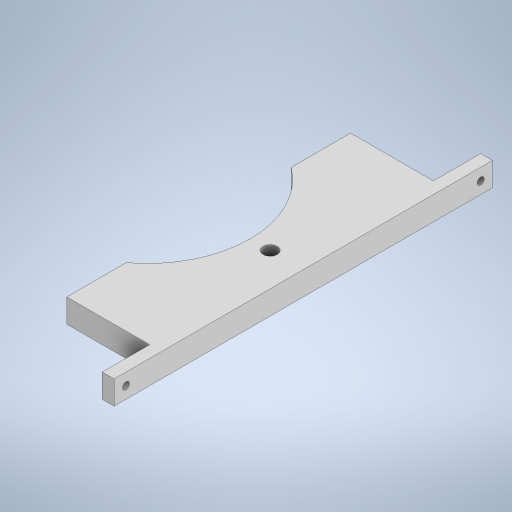
# Autodesk Inventor part: Мотор стенка
Saved by Autodesk Inventor 2023 (Build 270158000, 158)
## iProperties
Created: 2022-05-23
Part Number: Мотор стенка
Material: Типовые
Document SubType Name: Modeling
Designer: User
Density: 1 g/cm^3
Appearance: По умолчанию
Author: User
Autodesk Inventor part; units mm, degrees
ref_plane "YZ Plane" through (0, 0, 0) normal (1, 0, 0) x (0, 1, 0)
ref_plane "XZ Plane" through (0, 0, 0) normal (0, 1, 0) x (-1, 0, 0)
ref_plane "XY Plane" through (0, 0, 0) normal (0, 0, 1) x (1, 0, 0)
sketch "Эскиз1" plane through (0, 0, 0) normal (0, 1, 0) x (-1, 0, 0)
  line L0 (0, 0) -> (130, 0)
  line L1 (130, 0) -> (130, -120)
  line L2 (130, -120) -> (0, -120)
  line L3 (0, -120) -> (0, 0)
  line L4 (0, -60) -> (66, -60)
  circle A0 centre (66, -60) radius 43.5
  line L5 (130, 0) -> (90, 0)
  line L6 (90, -120) -> (130, -120)
  line L7 (130, -120) -> (130, 0)
  line L8 (0, 0) -> (40, 0)
  line L9 (40, 0) -> (40, -120)
  line L10 (40, -120) -> (0, -120)
  line L11 (0, -120) -> (0, 0)
  line L12 (0, 0) -> (0, 20)
  line L13 (0, 20) -> (5, 20)
  line L14 (5, 20) -> (5, -140)
  line L15 (5, -140) -> (0, -140)
  line L16 (0, -140) -> (0, -120)
  circle A1 centre (66, -60) radius 52
  circle A2 centre (14, -60) radius 3
  point P0 (40, -25.1252)
  point P1 (40, -94.8748)
  point P2 (5, -120)
  point P3 (5, 0)
  dimension "d34" = 104
  dimension "d0" = 130
  dimension "d1" = 120
  dimension "d2" = 66
  dimension "d16" = 87
  dimension "d20" = 40
  dimension "d21" = 20
  dimension "d22" = 5
  dimension "d23" = 160
  dimension "d35" = 6
  constraints: 34 end point, 6 perpendicular, 5 parallel, 4 horizontal, 3 point on line, 2 centre point, 1 coincident, 1 horizontal alignment, 1 midpoint, 1 vertical, 2 other
  measures "d0" distance of L1.end L2.end
  measures "d1" distance of L0.end L1.end
  measures "d2" distance of L4.start L4.end
  measures "d16" diameter of A0
  measures "d20" distance of L9.end L10.end
  measures "d21" distance of L0.start L12.end
  measures "d22" distance of L12.end L13.end
  measures "d23" distance of L13.end L14.end
  measures "d35" diameter of A2
extrude "Выдавливание1" add sketch "Эскиз1" along normal blind 10 contours L9 A1 A2 L4 L14 L0 | L14 L4 L3 L0 | L0 L12 L13 L14 | L9 A0 L4 A2 A1 | L14 L2 L3 L4 | L4 A2 A1 L9 L2 L14 | L14 L15 L16 L2 | A0 L9 A1 A2 L4
sketch "Эскиз2" plane through (-5, 0, 0) normal (-1, 0, 0) x (0, 0, 1)
  line L0 (20, 0) -> (20, 10) projected
  line L1 (20, 5) -> (15, 5)
  line L2 (-140, 0) -> (-140, 10) projected
  line L3 (-140, 5) -> (-135, 5)
  circle A0 centre (15, 5) radius 1.5
  circle A1 centre (-135, 5) radius 1.5
  point P0 (0, 0)
  dimension "d24" = 5
  dimension "d25" = 5
  dimension "d26" = 3
  dimension "d27" = 3
  constraints: 4 end point, 2 centre point, 2 coincident, 2 midpoint, 1 horizontal, 1 point on line
  measures "d24" distance of L1.start L1.end
  measures "d25" distance of L3.start L3.end
  measures "d26" diameter of A0
  measures "d27" diameter of A1
extrude "Выдавливание2" cut sketch "Эскиз2" against normal blind 19.5
thread "Резьба1" size "M3x0.5" class "6H" standard "ANSI Metric M Profile" full length
thread "Резьба2" size "M3x0.5" class "6H" standard "ANSI Metric M Profile" full length
